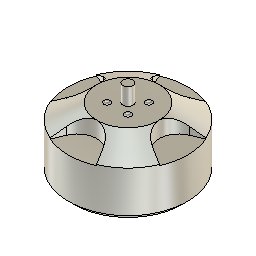
20021-022_motor (Autodesk Fusion 360 design; units mm, degrees)
Autodesk Fusion 360 part; units mm, degrees
sketch "Sketch1" plane through (0, 0, 0) normal (0, 0, 1) x (1, 0, 0)
  circle A0 centre (0, 0) radius 23.05
  line L0 (4.05, 4.05) -> (-4.05, 4.05) construction
  line L1 (-4.05, 4.05) -> (-4.05, -4.05) construction
  line L2 (-4.05, -4.05) -> (4.05, -4.05) construction
  line L3 (4.05, -4.05) -> (4.05, 4.05) construction
  line L4 (4.05, 4.05) -> (-4.05, -4.05) construction
  line L5 (-4.05, 4.05) -> (4.05, -4.05) construction
  circle A1 centre (0, 0) radius 1.95
  circle A2 centre (0, 0) radius 12
  line L6 (0, 0) -> (-9, -21.2203)
  line L7 (0, 0) -> (9, -21.2203)
  arc A3 (7.0767, -16.6855) -> (-7.0767, -16.6855) centre (0, -19.6868) ccw
  dimension "d1" = 46.1
  dimension "d2" = 8.1
  dimension "d3" = 8.1
  dimension "d4" = 3.9
  dimension "d5" = 24
  dimension "d19" = 18
  dimension "d20" = 9
  constraint coincident A0.centre A1.centre
  constraint perpendicular L0 L1
  constraint parallel L0 L2
  constraint parallel L1 L3
  constraint horizontal L0
  constraint coincident L4 A0.centre
  constraint coincident L5 A0.centre
  constraint coincident A0 L6.end
  constraint coincident A0 L7.end
  constraint tangent L7 A3
  constraint coincident L7 A3.start
  constraint coincident L6 A3.end
  constraint tangent L6 A3
  constraint tangent A2 A3
  measures "d1" diameter of A0
  measures "d2" distance of L1.end L2.end
  measures "d3" distance of L0.start L2.end
  measures "d4" diameter of A1
  measures "d5" diameter of A2
  measures "d19" distance of L6.end L7.end A0.centre
  measures "d20" horizontal distance of A0.centre L6.end
extrude "Extrude1" add sketch "Sketch1" against normal blind 23.8
chamfer "Chamfer1" distance 11 distance2 5.8 1 edges at (-21.4901, -8.3352, 0) measured on face at (5.3767, -4.1064, 0)
extrude "Extrude2" add sketch "Sketch1" along normal blind 6.6 contours A1 L6 L7 | A1 L6 L7
chamfer "Chamfer2" distance 2 angle 45 1 edges at (-21.4901, 8.3352, -23.8)
hole "Hole1" at (-4.05, -4.05, 0) at (-4.05, 4.05, 0) at (4.05, 4.05, 0) at (4.05, -4.05, 0) direction (0, 0, -1) diameter 2.529 depth 5 tip angle 180
thread "Thread1" "ISO Metric profile 3.0 M3x0.5 6H"
extrude "Extrude3" cut sketch "Sketch1" against normal up to surface (6.2 mm away) contours A0 L6 L7 A3
pattern_circular "C-Pattern1" count 4 over 360 about axis through (0, 0, 0) along (0, 0, 1) of "Extrude3"
equation "d9 = 23.8 mm - 18 mm"
equation "d20 = d19 / 2"
named bodies: "20021-022_motor"
